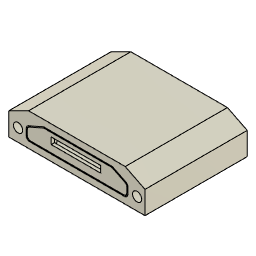
MicroSD Extension Mount (Autodesk Fusion 360 design; units mm, degrees)
Autodesk Fusion 360 part; units mm, degrees
ref_plane "WorkPlane1" through (0, 28, 0) normal (0, 1, 0) x (0, 0, 1)
sketch "Front Profile" plane through (0, 0, 0) normal (0, 1, 0) x (1, 0, 0)
  line L0 (0, 0) -> (28.2, 0)
  line L1 (0, 0) -> (0, -0.8)
  line L2 (0, -0.8) -> (28.2, -0.8)
  line L3 (28.2, 0) -> (28.2, -0.8)
  line L4 (0, -0.8) -> (6.25, -0.8) construction
  line L5 (6.25, -0.8) -> (21.25, -0.8)
  line L6 (21.25, -0.8) -> (21.25, -2.8)
  line L7 (21.25, -2.8) -> (6.25, -2.8)
  line L8 (6.25, -2.8) -> (6.25, -0.8)
  dimension "d1" = 28.2
  dimension "d2" = 0.8
  dimension "d3" = 6.25
  dimension "d4" = 15
  dimension "d5" = 2
  constraint coincident L0.start L1.start
  constraint horizontal L0
  constraint vertical L1
  constraint perpendicular L1 L2
  constraint perpendicular L2 L3
  constraint perpendicular L1 L4
  constraint horizontal L5
  constraint vertical L6
  constraint horizontal L7
  constraint vertical L8
  measures "d1" distance of L0.start L0.end
  measures "d2" distance of L0.start L1.end
  measures "d3" distance of L1.end L4.end
  measures "d4" distance of L4.end L5.end
  measures "d5" distance of L4.end L7.end
sketch "Sketch3" plane through (0, 0, 0) normal (0, 1, 0) x (1, 0, 0)
  line L0 (6.25, -0.8) -> (21.25, -0.8) construction
  line L1 (21.25, -0.8) -> (21.25, -2.8) construction
  line L2 (6.25, -2.8) -> (6.25, -0.8) construction
  line L3 (21.25, -2.8) -> (6.25, -2.8) construction
  line L4 (6, -0.55) -> (21.5, -0.55)
  line L5 (21.5, -0.55) -> (21.5, -3.05)
  line L6 (21.5, -3.05) -> (6, -3.05)
  line L7 (6, -3.05) -> (6, -0.55)
  line L8 (6.25, -2.8) -> (21.25, -2.8) construction
  line L9 (21.25, -2.8) -> (21.25, -0.8) construction
  line L10 (21.25, -0.8) -> (6.25, -0.8) construction
  line L11 (6.25, -0.8) -> (6.25, -2.8) construction
  line L12 (3.25, -5.8) -> (24.25, -5.8)
  line L13 (24.25, -5.8) -> (24.25, 2.2)
  line L14 (24.25, 2.2) -> (3.25, 2.2)
  line L15 (3.25, 2.2) -> (3.25, -5.8)
  line L16 (0, 0) -> (0, -0.8) construction
  line L17 (28.2, 0) -> (28.2, -0.8) construction
  line L18 (28.4, 0) -> (28.4, -0.8) construction
  line L19 (-0.2, 0) -> (-0.2, -0.8) construction
  dimension "d10" = -0.25
  dimension "d12" = -0.2
  dimension "d13" = 0.2
  constraint horizontal L8
  constraint vertical L9
  constraint horizontal L10
  constraint vertical L11
  constraint coincident L0.end L1.start
  constraint coincident L2.start L3.end
sketch "Back Profile" plane through (0, 28, 0) normal (0, 1, 0) x (1, 0, 0)
  line L0 (28.2, -0.8) -> (20.2, -0.8) construction
  line L1 (20.2, -0.8) -> (8.7, -0.8)
  line L2 (8.7, -0.8) -> (8.7, -2.8)
  line L3 (8.7, -2.8) -> (20.2, -2.8)
  line L4 (20.2, -2.8) -> (20.2, -0.8)
  line L5 (8.7, -0.8) -> (0, -0.8) construction
  line L6 (28.2, 0) -> (28.2, -0.8)
  line L7 (0, 0) -> (28.2, 0)
  line L8 (0, 0) -> (0, -0.8)
  line L9 (0, -0.8) -> (28.2, -0.8)
  dimension "d6" = 8
  dimension "d7" = 11.5
  dimension "d8" = 2
  constraint horizontal L1
  constraint vertical L2
  constraint horizontal L3
  constraint vertical L4
  measures "d6" distance of L0.start L0.end
  measures "d7" distance of L0.end L1.end
  measures "d8" distance of L0.end L3.end
ref_plane "WorkPlane2" through (0, 2, 0) normal (0, 1, 0) x (0, 0, 1)
sketch "Sketch5" plane through (0, 2, 0) normal (0, 1, 0) x (1, 0, 0)
  line L0 (28.2, 0) -> (28.2, -0.8) construction
  line L1 (0, 0) -> (28.2, 0) construction
  line L2 (0, 0) -> (0, -0.8) construction
  line L3 (0, -0.8) -> (28.2, -0.8)
  line L4 (0, -0.8) -> (5, -0.8)
  line L5 (5, -0.8) -> (5, 0)
  line L6 (28.2, -0.8) -> (23.7, -0.8)
  line L7 (23.7, -0.8) -> (23.7, 0)
  line L8 (21.25, -2.8) -> (6.25, -2.8) construction
  line L9 (21.25, -3) -> (6.25, -3)
  line L10 (5, -0.8) -> (5, -3)
  line L11 (6.25, -3) -> (5, -3)
  line L12 (21.25, -3) -> (23.7, -3)
  line L13 (23.7, -3) -> (23.7, -0.8)
  line L14 (23.7, -0.8) -> (21.25, -0.8)
  line L15 (0, -0.8) -> (28.2, -0.8) construction
  line L16 (28.2, -0.8) -> (28.2, 0.6)
  line L17 (28.2, 0.6) -> (0, 0.6)
  line L18 (0, 0.6) -> (0, -0.8)
  line L19 (4, -1.8) -> (4, -4)
  line L20 (6.25, -4) -> (4, -4)
  line L21 (21.25, -4) -> (6.25, -4)
  line L22 (21.25, -4) -> (24.7, -4)
  line L23 (24.7, -4) -> (24.7, -1.8)
  line L24 (29.2, -1.8) -> (29.2, 1.4)
  line L25 (29.2, 1.4) -> (-1, 1.4)
  line L26 (-1, 1.4) -> (-1, -1.8)
  line L27 (-1, -1.8) -> (4, -1.8)
  line L28 (24.7, -1.8) -> (29.2, -1.8)
  line L29 (5, 0) -> (5, 0.6)
  line L30 (23.7, 0) -> (23.7, 0.6)
  line L31 (4, -4) -> (-1, -1.8)
  line L32 (24.7, -4) -> (29.2, -1.8)
  dimension "d25" = 5
  dimension "d26" = 4.5
  dimension "d27" = 18.7
  dimension "d29" = 1.4
  constraint coincident L2.end L3.start
  constraint perpendicular L2 L4
  constraint coincident L1 L5.end
  constraint perpendicular L1 L5
  constraint coincident L0.end L3.end
  constraint perpendicular L0 L6
  constraint coincident L1 L7.end
  constraint perpendicular L1 L7
  constraint perpendicular L4 L10
  constraint perpendicular L10 L11
  constraint horizontal L12
  constraint vertical L13
  constraint horizontal L14
  constraint horizontal L15
  constraint vertical L16
  constraint horizontal L17
  constraint vertical L18
  constraint parallel L8 L9
  constraint parallel L16 L24
  constraint parallel L17 L25
  constraint parallel L18 L26
  constraint parallel L15 L27
  constraint collinear L27 L28
  constraint parallel L10 L19
  constraint parallel L11 L20
  constraint parallel L9 L21
  constraint parallel L12 L22
  constraint parallel L13 L23
  constraint coincident L17 L29.end
  constraint perpendicular L17 L29
  constraint coincident L17 L30.end
  constraint perpendicular L17 L30
  measures "d25" distance of L2.end L4.end
  measures "d26" distance of L0.end L6.end
  measures "d27" distance of L5 L7
  measures "d29" distance of L2.end L17.end
extrude "Extrude4" add sketch "Sketch5" against normal blind 2 contours L3 L4 L5 L17 L18 L29 | L3 L6 L7 L16 L17 L30 | L19 L20 L21 L22 L23 L24 L25 L26 L27 L28 | L19 L27 L31 | L23 L28 L32 makes body 1
sketch "Sketch6" plane through (0, 0, 0) normal (0, 1, 0) x (1, 0, 0)
  line L0 (5, -3) -> (23.7, -3)
  line L1 (23.7, -3) -> (23.7, 0.6)
  line L2 (23.7, 0.6) -> (5, 0.6)
  line L3 (5, 0.6) -> (5, -0.8)
  line L4 (5, -0.8) -> (5, -3)
  line L5 (24.7, -4) -> (4, -4)
  line L6 (-1, -1.8) -> (-1, 1.4)
  line L7 (-1, 1.4) -> (29.2, 1.4)
  line L8 (29.2, 1.4) -> (29.2, -1.8)
  line L9 (21.25, -0.8) -> (21.25, -2.8)
  line L10 (21.25, -2.8) -> (6.25, -2.8)
  line L11 (6.25, -0.8) -> (21.25, -0.8)
  line L12 (6.25, -2.8) -> (6.25, -0.8)
  line L13 (4, -4) -> (-1, -1.8)
  line L14 (24.7, -4) -> (29.2, -1.8)
  line L15 (4, -4) -> (-1, -1.8)
  line L16 (29.2, -1.8) -> (24.7, -4)
  constraint coincident L5.end L13.start
  constraint coincident L6.start L13.end
  constraint coincident L5.start L14.start
  constraint coincident L8.end L14.end
extrude "Extrude5" add sketch "Sketch6" against normal blind 1 contours L0 L1 L2 L3 L4 | L5 L6 L7 L8 L13 L14 L15 L16 bodies 1
extrude "Extrude6" add sketch "Sketch5" along normal blind 26 bodies 1
chamfer "Chamfer1" distance 0.6 angle 45 2 edges at (23.7, 15, 0.8) (5, 15, 0.8) on bodies 1
move_body "Move1" bodies 1 to x (1, 0, 0) y (0, 0, 1) z (0, -1, 0) at (0, 3, 5)
copy_body "Body->Comp1" bodies 1 removing the originals makes body 2 in component "MicroSD Extension - Inner Sleeve"
sketch "Sketch7" plane through (0, 28, 0) normal (0, 1, 0) x (1, 0, 0)
  line L0 (28.2, 0.6) -> (28.2, -0.8) construction
  line L1 (28.2, -0.8) -> (24.3, -0.8) construction
  line L2 (23.7, -1.4) -> (23.7, -3) construction
  line L3 (23.7, -3) -> (5, -3) construction
  line L4 (5, -3) -> (5, -1.4) construction
  line L5 (4.4, -0.8) -> (0, -0.8) construction
  line L6 (0, -0.8) -> (0, 0.6) construction
  line L7 (0, 0.6) -> (28.2, 0.6) construction
  line L8 (4, -4) -> (24.7, -4) construction
  line L9 (24.7, -4) -> (29.2, -1.8) construction
  line L10 (29.2, -1.8) -> (29.2, 1.4) construction
  line L11 (29.2, 1.4) -> (-1, 1.4) construction
  line L12 (-1, 1.4) -> (-1, -1.8) construction
  line L13 (-1, -1.8) -> (4, -4) construction
  line L14 (-1.3, 1.7) -> (-1.3, -1.9958)
  line L15 (-1.3, -1.9958) -> (3.9369, -4.3)
  line L16 (3.9369, -4.3) -> (24.7694, -4.3)
  line L17 (24.7694, -4.3) -> (29.5, -1.9873)
  line L18 (29.5, -1.9873) -> (29.5, 1.7)
  line L19 (29.5, 1.7) -> (-1.3, 1.7)
  line L20 (31.45, 3.65) -> (-3.25, 3.65)
  line L21 (-3.25, 3.65) -> (-3.25, -3.2682) construction
  line L22 (-3.25, -3.2682) -> (3.5269, -6.25) construction
  line L23 (3.5269, -6.25) -> (25.2206, -6.25)
  line L24 (25.2206, -6.25) -> (31.45, -3.2045) construction
  line L25 (31.45, -3.2045) -> (31.45, 3.65) construction
  line L26 (29.5, -0.1436) -> (32.3, -0.1436) construction
  circle A0 centre (32.3, -0.1436) radius 1.4
  line L27 (31.45, 3.65) -> (34.7, 3.65)
  line L28 (25.2206, -6.25) -> (28.7, -6.25)
  line L29 (-1, -0.2) -> (-3.8, -0.2) construction
  circle A1 centre (-3.8, -0.2) radius 1.4
  line L30 (34.7, -3.25) -> (34.7, 3.65)
  line L31 (34.7, -3.25) -> (28.7, -6.25)
  line L32 (-3.8, -0.2) -> (-6.6, -0.2) construction
  line L33 (-6.6, -0.2) -> (-6.6, 3.65) construction
  line L34 (-3.25, 3.65) -> (-6.6, 3.65)
  line L35 (3.5269, -6.25) -> (-0.6, -6.25)
  line L36 (-6.6, 3.65) -> (-6.6, -3.25)
  line L37 (-0.6, -6.25) -> (-6.6, -3.25)
  line L38 (23.7, -3) -> (5, -3)
  line L39 (5, -3) -> (5, 0.6)
  line L40 (5, 0.6) -> (23.7, 0.6)
  line L41 (23.7, 0.6) -> (23.7, -3)
  line L42 (5, -1.4) -> (4.4, -0.8)
  line L43 (24.3, -0.8) -> (23.7, -1.4)
  point P0 (34.7, -6.25)
  point P1 (-6.6, -6.25)
  dimension "d38" = 0.3
  dimension "d39" = 2.25
  dimension "d40" = 2.8
  dimension "d41" = 2.8
  dimension "d43" = 2.8
  dimension "d44" = 2.8
  dimension "d45" = 3
  dimension "d46" = 6
  dimension "d47" = 2.8
  dimension "d48" = 6
  dimension "d49" = 3
  constraint midpoint L18 L26.start
  constraint perpendicular L25 L26
  constraint coincident L26.end A0.centre
  constraint perpendicular L25 L27
  constraint parallel L23 L28
  constraint midpoint L12 L29.start
  constraint perpendicular L21 L29
  constraint coincident L29.end A1.centre
  constraint coincident P0 L30
  constraint coincident L28 P0
  constraint perpendicular L21 L32
  constraint perpendicular L32 L33
  constraint perpendicular L33 L34
  constraint parallel L23 L35
  constraint perpendicular L35 L36
  constraint coincident L35 P1
  constraint coincident P1 L36
  constraint horizontal L38
  constraint vertical L39
  constraint horizontal L40
  constraint vertical L41
  constraint coincident L7 L39.end
  constraint coincident L2.end L3.start
  measures "d40" diameter of A0
  measures "d41" distance of L26.start L26.end
  measures "d43" distance of L29.start L29.end
  measures "d44" diameter of A1
  measures "d45" distance of P0 L30.start
  measures "d46" distance of P0 L28.end
  measures "d47" distance of L29.end L32.end
  measures "d48" distance of P1 L35.end
  measures "d49" distance of P1 L36.end
extrude "Extrude1" add sketch "Sketch7" along normal blind 2 separate body contours L14 L15 L16 L17 L18 L19 | L20 L23 L27 L28 L30 L31 L34 L35 L36 L37 | A0 | A1 makes body 3 in component "MicroSD Extension - Outer Shell"
extrude "Extrude2" add sketch "Sketch7" against normal blind 29 contours L20 L23 L27 L28 L30 L31 L34 L35 L36 L37 | A0 | A1 bodies 3 in component "MicroSD Extension - Outer Shell"
extrude "Extrude3" cut sketch "Sketch7" along normal blind 6 from surface at -29 contours A0 | A1 bodies 3 in component "MicroSD Extension - Outer Shell"
move_body "Move1'" bodies 3 to x (1, 0, 0) y (0, 0, -1) z (0, 1, 0) at (0, 33.65, 26.35) in component "MicroSD Extension - Outer Shell"
fillet "Fillet1" radius 1 6 edges at (-1, 1.2, 18.5) (29.2, 1.2, 18.5) (24.7, -1, 18.5) (4, -1, 18.5) (-1, 4.4, 18.5) (29.2, 4.4, 18.5) on bodies 2 in component "MicroSD Extension - Inner Sleeve"
fillet "Fillet1'" radius 1 6 edges at (-1.3, 31.95, 12.85) (29.5, 31.95, 12.85) (29.5, 35.6373, 12.85) (24.7694, 37.95, 12.85) (-1.3, 35.6458, 12.85) (3.9369, 37.95, 12.85) on bodies 3 in component "MicroSD Extension - Outer Shell"
move_face "OffsetFaces1" offset -0.2 1 faces at (11.2333, 33.05, -2.9833) on bodies 3 in component "MicroSD Extension - Outer Shell"
move_face "OffsetFaces1'" offset -0.2 1 faces at (11.0667, 3.6, 24.3333) on bodies 2 in component "MicroSD Extension - Inner Sleeve"
component "MicroSD Extension - Inner Sleeve" placed x (1, 0, 0) y (0, 0, -1) z (0, 1, 0) at (0, -5, 3)
component "MicroSD Extension - Outer Shell" placed x (1, 0, 0) y (0, 0, 1) z (0, -1, 0) at (0, 26.35, -33.65)
